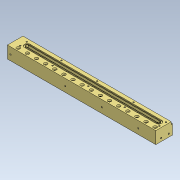
# Autodesk Inventor part: main_manifold_8v_v02
Saved by Autodesk Inventor 2022.4 (Build 264492010, 492A)
## iProperties
Created: 2021-03-09
Part Number: main_manifold_8v_v02
Material: Generic
Document SubType Name: Modeling
Designer: shann
Density: 1 g/cm^3
Appearance: Default(1)
propValve:hole_outlet:distanceFromBtm: 0.194 in
propValve:oring:depth: 0.055 in
propValve:hole_outlet:radius: 0.068 in
a_mainManifold:y:height: 0.800 in
a_mainManifold:z:width: 1.100 in
a_mainManifold:x:length: 9.750 in
flowSensor:hole_insert:diameter: 0.225 in
flowSensor:hole_insert:depth: 0.125 in
propValve:hole_outlet:dist_from_btm: 0.212 in
x_e1: 0.00 deg
propValve:d2: 0.281 in
propValve:d3: 0.145 in
propValve:hole_inlet:diameter: 0.136 in
propValve:hole_inlet:depth: 0.500 in
propValve:hole_outlet:diameter: 0.136 in
propValve:hole_outlet:depth: 0.915 in
propValve:440screws:diameter: 0.085 in
propValve:inlet_ycoord: 0.057 in
flowSensor:hole_insert:depth_max: 0.126 in
propValve:hole_inlet:radius: 0.068 in
a_mainInlet:y:distFromTop: 0.250 in
a_mainInlet:z:distToBack: 0.500 in
a_mainInlet:z:distToFront: 0.600 in
propValve:cutout:y: 0.160 in
propValve:cutout:z: 0.085 in
x_e2: 0.00 deg
bath:depth: 0.375 in
x_e3: 0.00 deg
x_e4: 0.00 deg
MMCscrews:x:distFromFlowSensor:L: 0.300 in
MMCscrews:distFromFront: 0.185 in
flowSensor:to_front_face: 0.185 in
d319: 0.300 in
d327: 3.500 in
d328: 2.500 in
d329: 2.500 in
bath:ID: 0.076 in
distance_between_MFCs: 1.200 in
bath:oring:space_from_bath: 0.025 in
flowSensor:hole:depth: 0.280 in
flowSensor:hole:diameter: 0.136 in
propValve:d0: 0.312 in
propValve:d1: 0.156 in
MPscrews:spacing:1: 3.600 in
MPscrews:spacing:2: 2.400 in
MPscrews:spacing:3: 2.400 in
screws:4_40:propValve:hole:depth: 0.300 in
screws:4_40:MMC:throughHole:head:depth: 0.112 in
screws:4_40:MMC:throughHole:head:diameter: 0.219 in
screws:4_40:MMC:throughHole:diameter: 0.129 in
bath:oring:gland_depth: 0.052 in
propValve:oring:OD: 0.245 in
propValve:oring:OD:outlet: 0.245 in
propValve:oring:OD:inlet: 0.245 in
propValve:oring:depth:inlet: 0.055 in
propValve:oring:depth:outlet: 0.055 in
screws:4_40:propValve:thread:depth: 0.250 in
bath:length: 8.650 in
oring_OD: 0.185 in
TCscrews:x:dist_from_bath:end:L: 0.245 in
TCscrews:z:dist_from_bath:end: 0.215 in
TCscrews:diameter_sketch: 0.129 in
TCscrews:z:dist_from_bath: 0.290 in
TCscrews:dist:1: 2.200 in
TCscrews:dist:2: 2.350 in
TCscrews:dist:3: 2.400 in
screws:4_40:TC:thread:depth: 0.175 in
screws:4_40:TC:hole:depth: 0.200 in
screws:4_40:MP:thread:depth: 0.250 in
screws:4_40:MP:hole:depth: 0.300 in
bath:dist_from_propValve_left: 0.125 in
MPscrews:dist_from_btm: 0.357 in
MPscrews:dist_from_edge_left: 0.200 in
TCscrews:dist:total: 9.150 in
mainInlet:tube:diameter: 0.250 in
mainInlet:tube:depth: 0.701 in
mountingScrews:dist_from_btm: 0.200 in
screws:4_40:mountingScrews:thread:depth:1: 0.250 in
screws:4_40:mountingScrews:hole:depth:1: 0.300 in
mountingScrews:dist_between: 0.500 in
screws:4_40:mountingScrews:thread:depth:2: 0.250 in
screws:4_40:mountingScrews:hole:depth:2: 0.300 in
mainInlet_fitting:hole:depth: 0.300 in
bath:oring:gland_width: 0.084 in
mainInlet:tube:radius: 0.125 in
oring_ID: 0.101 in
MPscrews:spacing:total: 8.400 in
TCscrews:x:dist_from_bath:end:R: 0.255 in
TCscrews:dist:4: 2.200 in
bath:dist_from_propValve_right: 0.125 in
TCscrews:x:dist_from_end: 0.145 in
mountingScrews:dist_from_front: 0.350 in
mountingScrews:dist_from_back: 0.250 in
propValve:x:distFromLeft: 0.825 in
d439: 0.000 in
screws:4_40:MP:thread:depth:2: 0.250 in
screws:4_40:MP:hole:depth:2: 0.300 in
Author: shann
Autodesk Inventor part; units mm, degrees
ref_plane "YZ Plane" through (0, 0, 0) normal (1, 0, 0) x (0, 1, 0)
ref_plane "XZ Plane" through (0, 0, 0) normal (0, 1, 0) x (-1, 0, 0)
ref_plane "XY Plane" through (0, 0, 0) normal (0, 0, 1) x (1, 0, 0)
sketch "Sketch:MM: main inlet" plane through (0, 0, 0) normal (1, 0, 0) x (0, 1, 0)
  line L0 (20.32, 0) -> (0, 0)
  line L1 (0, 0) -> (0, -27.94)
  line L2 (0, -27.94) -> (20.32, -27.94)
  line L3 (20.32, -27.94) -> (20.32, 0)
  point P0 (13.97, -15.24)
  constraints: 8 end point, 3 perpendicular, 1 coincident, 1 horizontal alignment, 1 vertical, 1 vertical alignment, 3 other
extrude "Ex: main" add sketch "Sketch:MM: main inlet" along normal blind 247.65
hole "Hole: main inlet: 1/8\" NPT thread" at (0, 13.97, -15.24) direction (1, 0, 0) diameter 7.9502 depth 7.62 taper from width 8.7366 to width 8.304 over 6.924 thread size "1/8" designation "1/8 - 27 NPT" standard "NPT"
hole "Hole: main inlet: tube" at (0, 13.97, -15.24) direction (1, 0, 0) diameter 6.35 depth 17.8054
sketch "Sketch:MM: prop valves" plane through (0, 0, -27.94) normal (0, 0, -1) x (-1, 0, 0)
  line L0 (-16.9926, 9.0678) -> (-24.9174, 9.0678) construction
  line L1 (-47.4726, 9.0678) -> (-55.3974, 9.0678) construction
  line L2 (-77.9526, 9.0678) -> (-85.8774, 9.0678) construction
  line L3 (-108.4326, 9.0678) -> (-116.3574, 9.0678) construction
  line L4 (-138.9126, 9.0678) -> (-146.8374, 9.0678) construction
  line L5 (-169.3926, 9.0678) -> (-177.3174, 9.0678) construction
  line L6 (-199.8726, 9.0678) -> (-207.7974, 9.0678) construction
  line L7 (-230.3526, 9.0678) -> (-238.2774, 9.0678) construction
  line L8 (-47.4726, 9.0678) -> (-51.435, 5.3848) construction
  line L9 (-16.9926, 9.0678) -> (-20.955, 5.3848) construction
  line L10 (-77.9526, 9.0678) -> (-81.915, 5.3848) construction
  line L11 (-169.3926, 9.0678) -> (-173.355, 5.3848) construction
  line L12 (-199.8726, 9.0678) -> (-203.835, 5.3848) construction
  line L13 (-230.3526, 9.0678) -> (-234.315, 5.3848) construction
  line L14 (-138.9126, 9.0678) -> (-142.875, 5.3848) construction
  line L15 (-108.4326, 9.0678) -> (-112.395, 5.3848) construction
  line L16 (-20.955, 12.5222) -> (-51.435, 12.5222) construction
  line L17 (-51.435, 12.5222) -> (-81.915, 12.5222) construction
  line L18 (-81.915, 12.5222) -> (-112.395, 12.5222) construction
  line L19 (-112.395, 12.5222) -> (-142.875, 12.5222) construction
  line L20 (-142.875, 12.5222) -> (-173.355, 12.5222) construction
  line L21 (-173.355, 12.5222) -> (-203.835, 12.5222) construction
  line L22 (-203.835, 12.5222) -> (-234.315, 12.5222) construction
  point P0 (0, 0)
  point P1 (0, 13.97)
  dimension "distance_between_MFCs" = 30.48
  constraints: 46 end point, 30 horizontal alignment, 20 equal length, 9 vertical alignment, 5 other
  measures "distance_between_MFCs" distance of L16.start L16.end
sketch "Sketch:MM: prop valve cutout" plane through (0, 0, 0) normal (1, 0, 0) x (0, 1, 0)
  line L0 (20.32, -27.94) -> (20.32, 0) projected
  line L1 (0, -27.94) -> (20.32, -27.94) projected
  line L2 (20.32, -25.781) -> (16.256, -25.781)
  line L3 (16.256, -25.781) -> (16.256, -27.94)
  point P0 (0, 0)
  point P1 (12.5222, -27.94)
  constraints: 4 end point, 2 perpendicular, 2 point on line, 1 horizontal alignment, 1 vertical alignment
hole "Hole: propValve: inlet" at (20.955, 12.5222, -27.94) at (51.435, 12.5222, -27.94) at (81.915, 12.5222, -27.94) at (112.395, 12.5222, -27.94) at (142.875, 12.5222, -27.94) at (173.355, 12.5222, -27.94) at (203.835, 12.5222, -27.94) at (234.315, 12.5222, -27.94) direction (0, 0, 1) diameter 3.4544 depth 12.7 counterbore diameter 6.223 counterbore depth 1.397
hole "Hole: propValve: outlet" at (20.955, 5.3848, -27.94) at (51.435, 5.3848, -27.94) at (81.915, 5.3848, -27.94) at (112.395, 5.3848, -27.94) at (142.875, 5.3848, -27.94) at (173.355, 5.3848, -27.94) at (203.835, 5.3848, -27.94) at (234.315, 5.3848, -27.94) direction (0, 0, 1) diameter 3.4544 depth 23.241 counterbore diameter 6.223 counterbore depth 1.397
hole "Hole: propValve: 4-40 thread" at (24.9174, 9.0678, -27.94) at (16.9926, 9.0678, -27.94) at (47.4726, 9.0678, -27.94) at (55.3974, 9.0678, -27.94) at (77.9526, 9.0678, -27.94) at (85.8774, 9.0678, -27.94) at (108.4326, 9.0678, -27.94) at (116.3574, 9.0678, -27.94) at (138.9126, 9.0678, -27.94) at (146.8374, 9.0678, -27.94) at (169.3926, 9.0678, -27.94) at (177.3174, 9.0678, -27.94) at (199.8726, 9.0678, -27.94) at (207.7974, 9.0678, -27.94) at (230.3526, 9.0678, -27.94) at (238.2774, 9.0678, -27.94) direction (0, 0, 1) diameter 2.1565 depth 7.62 thread size "4-40 UNC" class "2B" standard "ANSI Unified Screw Threads"
extrude "Ex: prop valve cutout" cut sketch "Sketch:MM: prop valve cutout" along normal through all
sketch "Sketch:MM: flow sensor" plane through (0, 0, -27.94) normal (0, -1, 0) x (1, 0, 0)
  line L0 (19.2278, 23.241) -> (22.6822, 23.241) projected
  line L1 (49.7078, 23.241) -> (53.1622, 23.241) projected
  line L2 (110.6678, 23.241) -> (114.1222, 23.241) projected
  line L3 (80.1878, 23.241) -> (83.6422, 23.241) projected
  line L4 (141.1478, 23.241) -> (144.6022, 23.241) projected
  line L5 (171.6278, 23.241) -> (175.0822, 23.241) projected
  line L6 (202.1078, 23.241) -> (205.5622, 23.241) projected
  line L7 (232.5878, 23.241) -> (236.0422, 23.241) projected
  line L8 (0, 27.94) -> (247.65, 27.94) projected
  point P0 (20.955, 23.241)
  point P1 (51.435, 23.241)
  point P2 (51.435, 23.241)
  point P3 (20.955, 23.241)
  point P4 (81.915, 23.241)
  point P5 (112.395, 23.241)
  point P6 (81.915, 23.241)
  point P7 (112.395, 23.241)
  point P8 (142.875, 23.241)
  point P9 (173.355, 23.241)
  point P10 (203.835, 23.241)
  point P11 (234.315, 23.241)
  point P12 (142.875, 23.241)
  point P13 (173.355, 23.241)
  point P14 (203.835, 23.241)
  point P15 (234.315, 23.241)
  constraints: 8 coincident, 8 midpoint, 1 other
sketch "Sketch:MM: MMC screws" plane through (0, 20.32, 0) normal (0, 1, 0) x (1, 0, 0)
  line L0 (0, 0) -> (0, 27.94) projected
  line L1 (43.815, 4.699) -> (59.055, 4.699) construction
  line L2 (0, 0) -> (247.65, 0) projected
  line L3 (13.335, 4.699) -> (28.575, 4.699) construction
  line L4 (74.295, 4.699) -> (89.535, 4.699) construction
  line L5 (104.775, 4.699) -> (120.015, 4.699) construction
  line L6 (135.255, 4.699) -> (150.495, 4.699) construction
  line L7 (165.735, 4.699) -> (180.975, 4.699) construction
  line L8 (196.215, 4.699) -> (211.455, 4.699) construction
  line L9 (226.695, 4.699) -> (241.935, 4.699) construction
  point P0 (20.955, 4.699)
  point P1 (112.395, 4.699)
  point P2 (51.435, 4.699)
  point P3 (81.915, 4.699)
  point P4 (0, 25.781)
  point P5 (0, 25.781)
  point P6 (0, 25.781)
  point P7 (142.875, 4.699)
  point P8 (173.355, 4.699)
  point P9 (203.835, 4.699)
  point P10 (234.315, 4.699)
  point P11 (20.955, 4.699)
  point P12 (51.435, 4.699)
  point P13 (81.915, 4.699)
  point P14 (112.395, 4.699)
  point P15 (142.875, 4.699)
  point P16 (173.355, 4.699)
  point P17 (203.835, 4.699)
  point P18 (234.315, 4.699)
  dimension "d319" = 7.62
  constraints: 24 coincident, 16 end point, 8 horizontal, 8 midpoint, 7 collinear, 1 horizontal alignment, 1 other
  measures "d319" distance of point (28.575, 4.699) point (20.955, 4.699)
hole "Hole: flowSensor" at (20.955, 0, -4.699) at (51.435, 0, -4.699) at (81.915, 0, -4.699) at (112.395, 0, -4.699) at (142.875, 0, -4.699) at (173.355, 0, -4.699) at (203.835, 0, -4.699) at (234.315, 0, -4.699) direction (0, 1, 0) diameter 3.4544 depth 7.112 counterbore diameter 5.715 counterbore depth 3.175
hole "Hole: MMC screws: 4-40 through hole" at (13.335, 20.32, -4.699) at (43.815, 20.32, -4.699) at (59.055, 20.32, -4.699) at (28.575, 20.32, -4.699) at (74.295, 20.32, -4.699) at (89.535, 20.32, -4.699) at (104.775, 20.32, -4.699) at (120.015, 20.32, -4.699) at (135.255, 20.32, -4.699) at (150.495, 20.32, -4.699) at (165.735, 20.32, -4.699) at (180.975, 20.32, -4.699) at (196.215, 20.32, -4.699) at (211.455, 20.32, -4.699) at (226.695, 20.32, -4.699) at (241.935, 20.32, -4.699) direction (0, -1, 0) diameter 3.2766 end through all counterbore diameter 5.5626 counterbore depth 2.8448 clearance for "Socket Head Cap Screw" size "#4" standard "Ansi Unified Screw Threads"
sketch "Sketch:MM: bath & TC screws" plane through (0, 20.32, 0) normal (0, 1, 0) x (1, 0, 0)
  arc A0 (17.78, 17.1704) -> (17.78, 13.3096) centre (17.78, 15.24) ccw
  arc A1 (237.49, 13.3096) -> (237.49, 17.1704) centre (237.49, 15.24) ccw
  line L0 (17.78, 13.3096) -> (237.49, 13.3096)
  line L1 (17.78, 17.1704) -> (237.49, 17.1704)
  arc A2 (17.78, 17.8054) -> (17.78, 12.6746) centre (17.78, 15.24) ccw
  arc A3 (237.49, 12.6746) -> (237.49, 17.8054) centre (237.49, 15.24) ccw
  line L2 (17.78, 12.6746) -> (237.49, 12.6746)
  line L3 (17.78, 17.8054) -> (237.49, 17.8054)
  arc A4 (17.78, 19.939) -> (17.78, 10.541) centre (17.78, 15.24) ccw
  arc A5 (237.49, 10.541) -> (237.49, 19.939) centre (237.49, 15.24) ccw
  line L4 (237.49, 19.939) -> (17.78, 19.939)
  line L5 (237.49, 10.541) -> (17.78, 10.541)
  line L6 (0, 27.94) -> (247.65, 27.94) projected
  line L7 (11.557, 20.701) -> (11.557, 9.779) construction
  line L8 (67.437, 22.606) -> (67.437, 7.874) construction
  circle A6 centre (11.557, 20.701) radius 1.6383 construction
  circle A7 centre (11.557, 9.779) radius 1.6383 construction
  circle A8 centre (243.967, 20.701) radius 1.6383 construction
  circle A9 centre (243.967, 9.779) radius 1.6383 construction
  point P0 (0, 0)
  point P1 (20.955, 27.94)
  point P2 (234.315, 27.94)
  point P3 (127.127, 22.606)
  point P4 (127.127, 7.874)
  point P5 (188.087, 22.606)
  point P6 (188.087, 7.874)
  point P7 (11.557, 15.24)
  point P8 (11.557, 15.24)
  point P9 (67.437, 15.24)
  point P10 (67.437, 15.24)
  point P11 (0, 15.24)
  dimension "oring_ID" = 2.5654
  dimension "oring_OD" = 4.699
  constraints: 16 end point, 14 horizontal alignment, 12 point on circle, 10 centre point, 10 coincident, 9 tangent, 7 vertical alignment, 5 equal radius, 4 parallel, 2 midpoint, 1 concentric, 1 horizontal, 9 other
  measures "oring_ID" radius of A2
  measures "oring_OD" radius of A4
extrude "Ex: bath" cut sketch "Sketch:MM: bath & TC screws" against normal blind 9.525 contours L1 A1 L0 A0
extrude "Ex: bath: o-ring" cut sketch "Sketch:MM: bath & TC screws" against normal blind 1.3208 contours L4 A5 L5 A4
hole "Hole: TC screws: 4-40 thread" at (243.967, 20.32, -20.701) at (243.967, 20.32, -9.779) at (127.127, 20.32, -22.606) at (127.127, 20.32, -7.874) at (67.437, 20.32, -22.606) at (67.437, 20.32, -7.874) at (11.557, 20.32, -20.701) at (11.557, 20.32, -9.779) at (188.087, 20.32, -22.606) at (188.087, 20.32, -7.874) direction (0, -1, 0) diameter 2.1565 depth 5.08 thread size "4-40 UNC" class "2B" standard "ANSI Unified Screw Threads"
sketch "Sketch:MM: MP screws" plane through (0, 0, 0) normal (0, 0, 1) x (1, 0, 0)
  point P0 (0, 0)
  point P1 (5.08, 9.0678)
  point P2 (218.44, 9.0678)
  point P3 (96.52, 9.0678)
  point P4 (157.48, 9.0678)
  constraints: 7 horizontal alignment, 2 other
sketch "Sketch:MM: MP screws:2" plane through (247.65, 0, -27.94) normal (0, 0, -1) x (-1, 0, 0)
  point P0 (247.65, 0)
  point P1 (29.21, 9.0678)
  point P2 (90.17, 9.0678)
  point P3 (242.57, 9.0678)
  point P4 (151.13, 9.0678)
hole "Hole: MP screws: 4-40 thread" at (218.44, 9.0678, 0) at (157.48, 9.0678, 0) at (96.52, 9.0678, 0) at (5.08, 9.0678, 0) direction (0, 0, -1) diameter 2.1565 depth 7.62 thread size "4-40 UNC" class "2B" standard "ANSI Unified Screw Threads"
hole "Hole: MP screws: 4-40 thread:2" at (157.48, 9.0678, -27.94) at (218.44, 9.0678, -27.94) at (96.52, 9.0678, -27.94) at (5.08, 9.0678, -27.94) direction (0, 0, 1) diameter 2.1565 depth 7.62 thread size "4-40 UNC" class "2B" standard "ANSI Unified Screw Threads"
sketch "Sketch:MM: mounting screws:1" plane through (0, 0, 0) normal (-1, 0, 0) x (0, 0, 1)
  line L0 (-27.94, 0) -> (-27.94, 16.256) projected
  line L1 (-21.59, 5.08) -> (-8.89, 5.08) construction
  point P0 (0, 0)
  point P1 (-15.24, 13.97)
  point P2 (-15.24, 5.08)
  constraints: 2 coincident, 2 end point, 2 horizontal alignment, 1 midpoint, 1 vertical alignment, 3 other
sketch "Sketch:MM: mounting screws:2" plane through (247.65, 0, 0) normal (1, 0, 0) x (0, 0, -1)
  point P0 (0, 0)
  point P1 (21.59, 5.08)
  point P2 (8.89, 5.08)
hole "Hole: mounting screws:1: 4-40 thread" at (0, 5.08, -21.59) at (0, 5.08, -8.89) direction (1, 0, 0) diameter 2.1565 depth 7.62 thread size "4-40 UNC" class "2B" standard "ANSI Unified Screw Threads"
hole "Hole: mounting screws:2: 4-40 thread" at (247.65, 5.08, -8.89) at (247.65, 5.08, -21.59) direction (-1, 0, 0) diameter 2.1565 depth 7.62 thread size "4-40 UNC" class "2B" standard "ANSI Unified Screw Threads"
ref_plane "MM front face" through (0, 0, 0) normal (0, 0, 1) x (1, 0, 0)
body "Solid1"
